Autodesk Inventor part; units mm, degrees
(part 2 of 2)
sketch "Sketch11" plane through (0, 0, 0) normal (0, -1, 0) x (1, 0, 0)
  arc A0 (-20.4663, -10.3703) -> (-20.3393, -10.1987) centre (-21.202, -9.693) ccw projected
  line L0 (-20.4663, -10.3703) -> (-19.459, -11.1159) projected
  arc A1 (-20.4246, -11.8044) -> (-19.459, -11.1159) centre (-21.202, -9.693) ccw projected
  line L1 (-20.4246, -11.8044) -> (-20.8013, -10.6092) projected
  arc A2 (-21.0049, -10.6734) -> (-20.8013, -10.6092) centre (-21.202, -9.693) ccw projected
  line L2 (-21.0049, -10.6734) -> (-20.6282, -11.8686) projected
  arc A3 (-21.8141, -11.8581) -> (-20.6282, -11.8686) centre (-21.202, -9.693) ccw projected
  line L3 (-21.8141, -11.8581) -> (-21.4164, -10.6698) projected
  arc A4 (-21.6188, -10.602) -> (-21.4164, -10.6698) centre (-21.202, -9.693) ccw projected
  line L4 (-21.6188, -10.602) -> (-22.0166, -11.7904) projected
  arc A5 (-22.9699, -11.0848) -> (-22.0166, -11.7904) centre (-21.202, -9.693) ccw projected
  line L5 (-22.9699, -11.0848) -> (-21.9495, -10.3572) projected
  arc A6 (-22.0735, -10.1834) -> (-21.9495, -10.3572) centre (-21.202, -9.693) ccw projected
  line L6 (-22.0735, -10.1834) -> (-23.0938, -10.911) projected
  arc A7 (-23.4503, -9.7799) -> (-23.0938, -10.911) centre (-21.202, -9.693) ccw projected
  line L7 (-23.4503, -9.7799) -> (-22.1972, -9.791) projected
  arc A8 (-22.1953, -9.5775) -> (-22.1972, -9.791) centre (-21.202, -9.693) ccw projected
  line L8 (-22.1953, -9.5775) -> (-23.4484, -9.5664) projected
  arc A9 (-23.072, -8.4418) -> (-23.4484, -9.5664) centre (-21.202, -9.693) ccw projected
  line L9 (-23.072, -8.4418) -> (-22.0647, -9.1873) projected
  arc A10 (-21.9377, -9.0157) -> (-22.0647, -9.1873) centre (-21.202, -9.693) ccw projected
  line L10 (-21.9377, -9.0157) -> (-22.945, -8.2701) projected
  arc A11 (-21.9794, -7.5816) -> (-22.945, -8.2701) centre (-21.202, -9.693) ccw projected
  line L11 (-21.9794, -7.5816) -> (-21.6027, -8.7768) projected
  arc A12 (-21.3991, -8.7126) -> (-21.6027, -8.7768) centre (-21.202, -9.693) ccw projected
  line L12 (-21.3991, -8.7126) -> (-21.7758, -7.5174) projected
  arc A13 (-20.5899, -7.5279) -> (-21.7758, -7.5174) centre (-21.202, -9.693) ccw projected
  line L13 (-20.5899, -7.5279) -> (-20.9876, -8.7162) projected
  arc A14 (-20.7852, -8.784) -> (-20.9876, -8.7162) centre (-21.202, -9.693) ccw projected
  line L14 (-20.7852, -8.784) -> (-20.3874, -7.5956) projected
  arc A15 (-19.4341, -8.3012) -> (-20.3874, -7.5956) centre (-21.202, -9.693) ccw projected
  line L15 (-19.4341, -8.3012) -> (-20.4545, -9.0288) projected
  arc A16 (-20.3305, -9.2026) -> (-20.4545, -9.0288) centre (-21.202, -9.693) ccw projected
  line L16 (-20.3305, -9.2026) -> (-19.3102, -8.475) projected
  arc A17 (-18.9537, -9.6061) -> (-19.3102, -8.475) centre (-21.202, -9.693) ccw projected
  line L17 (-18.9537, -9.6061) -> (-20.2068, -9.595) projected
  arc A18 (-20.2087, -9.8085) -> (-20.2068, -9.595) centre (-21.202, -9.693) ccw projected
  line L18 (-20.2087, -9.8085) -> (-18.9556, -9.8196) projected
  arc A19 (-19.332, -10.9442) -> (-18.9556, -9.8196) centre (-21.202, -9.693) ccw projected
  line L19 (-19.332, -10.9442) -> (-20.3393, -10.1987) projected
  circle A20 centre (0, 28.15) radius 6.2 projected
  arc A21 (20.3393, -10.1987) -> (20.4663, -10.3703) centre (21.202, -9.693) ccw projected
  line L20 (19.332, -10.9442) -> (20.3393, -10.1987) projected
  arc A22 (18.9556, -9.8196) -> (19.332, -10.9442) centre (21.202, -9.693) ccw projected
  line L21 (20.2087, -9.8085) -> (18.9556, -9.8196) projected
  arc A23 (20.2068, -9.595) -> (20.2087, -9.8085) centre (21.202, -9.693) ccw projected
  line L22 (18.9537, -9.6061) -> (20.2068, -9.595) projected
  arc A24 (19.3102, -8.475) -> (18.9537, -9.6061) centre (21.202, -9.693) ccw projected
  line L23 (20.3305, -9.2026) -> (19.3102, -8.475) projected
  arc A25 (20.4545, -9.0288) -> (20.3305, -9.2026) centre (21.202, -9.693) ccw projected
  line L24 (19.4341, -8.3012) -> (20.4545, -9.0288) projected
  arc A26 (20.3874, -7.5956) -> (19.4341, -8.3012) centre (21.202, -9.693) ccw projected
  line L25 (20.7852, -8.784) -> (20.3874, -7.5956) projected
  arc A27 (20.9876, -8.7162) -> (20.7852, -8.784) centre (21.202, -9.693) ccw projected
  line L26 (20.5899, -7.5279) -> (20.9876, -8.7162) projected
  arc A28 (21.7758, -7.5174) -> (20.5899, -7.5279) centre (21.202, -9.693) ccw projected
  line L27 (21.3991, -8.7126) -> (21.7758, -7.5174) projected
  arc A29 (21.6027, -8.7768) -> (21.3991, -8.7126) centre (21.202, -9.693) ccw projected
  line L28 (21.9794, -7.5816) -> (21.6027, -8.7768) projected
  arc A30 (22.945, -8.2701) -> (21.9794, -7.5816) centre (21.202, -9.693) ccw projected
  line L29 (21.9377, -9.0157) -> (22.945, -8.2701) projected
  arc A31 (22.0647, -9.1873) -> (21.9377, -9.0157) centre (21.202, -9.693) ccw projected
  line L30 (23.072, -8.4418) -> (22.0647, -9.1873) projected
  arc A32 (23.4484, -9.5664) -> (23.072, -8.4418) centre (21.202, -9.693) ccw projected
  line L31 (22.1953, -9.5775) -> (23.4484, -9.5664) projected
  arc A33 (22.1972, -9.791) -> (22.1953, -9.5775) centre (21.202, -9.693) ccw projected
  line L32 (23.4503, -9.7799) -> (22.1972, -9.791) projected
  arc A34 (23.0938, -10.911) -> (23.4503, -9.7799) centre (21.202, -9.693) ccw projected
  line L33 (22.0735, -10.1834) -> (23.0938, -10.911) projected
  arc A35 (21.9495, -10.3572) -> (22.0735, -10.1834) centre (21.202, -9.693) ccw projected
  line L34 (22.9699, -11.0848) -> (21.9495, -10.3572) projected
  arc A36 (22.0166, -11.7904) -> (22.9699, -11.0848) centre (21.202, -9.693) ccw projected
  line L35 (21.6188, -10.602) -> (22.0166, -11.7904) projected
  arc A37 (21.4164, -10.6698) -> (21.6188, -10.602) centre (21.202, -9.693) ccw projected
  line L36 (21.8141, -11.8581) -> (21.4164, -10.6698) projected
  arc A38 (20.6282, -11.8686) -> (21.8141, -11.8581) centre (21.202, -9.693) ccw projected
  line L37 (21.0049, -10.6734) -> (20.6282, -11.8686) projected
  arc A39 (20.8013, -10.6092) -> (21.0049, -10.6734) centre (21.202, -9.693) ccw projected
  line L38 (20.4246, -11.8044) -> (20.8013, -10.6092) projected
  arc A40 (19.459, -11.1159) -> (20.4246, -11.8044) centre (21.202, -9.693) ccw projected
  line L39 (20.4663, -10.3703) -> (19.459, -11.1159) projected
  arc A41 (-20.3393, -25.0623) -> (-20.4663, -24.8907) centre (-21.202, -25.568) ccw projected
  line L40 (-19.332, -24.3168) -> (-20.3393, -25.0623) projected
  arc A42 (-18.9556, -25.4414) -> (-19.332, -24.3168) centre (-21.202, -25.568) ccw projected
  line L41 (-20.2087, -25.4525) -> (-18.9556, -25.4414) projected
  arc A43 (-20.2068, -25.666) -> (-20.2087, -25.4525) centre (-21.202, -25.568) ccw projected
  line L42 (-18.9537, -25.6549) -> (-20.2068, -25.666) projected
  arc A44 (-19.3102, -26.786) -> (-18.9537, -25.6549) centre (-21.202, -25.568) ccw projected
  line L43 (-20.3305, -26.0584) -> (-19.3102, -26.786) projected
  arc A45 (-20.4545, -26.2322) -> (-20.3305, -26.0584) centre (-21.202, -25.568) ccw projected
  line L44 (-19.4341, -26.9598) -> (-20.4545, -26.2322) projected
  arc A46 (-20.3874, -27.6654) -> (-19.4341, -26.9598) centre (-21.202, -25.568) ccw projected
  line L45 (-20.7852, -26.477) -> (-20.3874, -27.6654) projected
  arc A47 (-20.9876, -26.5448) -> (-20.7852, -26.477) centre (-21.202, -25.568) ccw projected
  line L46 (-20.5899, -27.7331) -> (-20.9876, -26.5448) projected
  arc A48 (-21.7758, -27.7436) -> (-20.5899, -27.7331) centre (-21.202, -25.568) ccw projected
  line L47 (-21.3991, -26.5484) -> (-21.7758, -27.7436) projected
  arc A49 (-21.6027, -26.4842) -> (-21.3991, -26.5484) centre (-21.202, -25.568) ccw projected
  line L48 (-21.9794, -27.6794) -> (-21.6027, -26.4842) projected
  arc A50 (-22.945, -26.9909) -> (-21.9794, -27.6794) centre (-21.202, -25.568) ccw projected
  line L49 (-21.9377, -26.2453) -> (-22.945, -26.9909) projected
  arc A51 (-22.0647, -26.0737) -> (-21.9377, -26.2453) centre (-21.202, -25.568) ccw projected
  line L50 (-23.072, -26.8192) -> (-22.0647, -26.0737) projected
  arc A52 (-23.4484, -25.6946) -> (-23.072, -26.8192) centre (-21.202, -25.568) ccw projected
  line L51 (-22.1953, -25.6835) -> (-23.4484, -25.6946) projected
  arc A53 (-22.1972, -25.47) -> (-22.1953, -25.6835) centre (-21.202, -25.568) ccw projected
  line L52 (-23.4503, -25.4811) -> (-22.1972, -25.47) projected
  arc A54 (-23.0938, -24.35) -> (-23.4503, -25.4811) centre (-21.202, -25.568) ccw projected
  line L53 (-22.0735, -25.0776) -> (-23.0938, -24.35) projected
  arc A55 (-21.9495, -24.9038) -> (-22.0735, -25.0776) centre (-21.202, -25.568) ccw projected
  line L54 (-22.9699, -24.1762) -> (-21.9495, -24.9038) projected
  arc A56 (-22.0166, -23.4706) -> (-22.9699, -24.1762) centre (-21.202, -25.568) ccw projected
  line L55 (-21.6188, -24.659) -> (-22.0166, -23.4706) projected
  arc A57 (-21.4164, -24.5912) -> (-21.6188, -24.659) centre (-21.202, -25.568) ccw projected
  line L56 (-21.8141, -23.4029) -> (-21.4164, -24.5912) projected
  arc A58 (-20.6282, -23.3924) -> (-21.8141, -23.4029) centre (-21.202, -25.568) ccw projected
  line L57 (-21.0049, -24.5876) -> (-20.6282, -23.3924) projected
  arc A59 (-20.8013, -24.6518) -> (-21.0049, -24.5876) centre (-21.202, -25.568) ccw projected
  line L58 (-20.4246, -23.4566) -> (-20.8013, -24.6518) projected
  arc A60 (-19.459, -24.1451) -> (-20.4246, -23.4566) centre (-21.202, -25.568) ccw projected
  line L59 (-20.4663, -24.8907) -> (-19.459, -24.1451) projected
  circle A61 centre (30.16, -30.16) radius 2.2 projected
  circle A62 centre (-30.16, -30.16) radius 2.2 projected
  line L60 (46.4, 46.4) -> (46.4, -46.4) projected
  line L61 (-46.4, 46.4) -> (46.4, 46.4) projected
  line L62 (-46.4, -46.4) -> (-46.4, 46.4) projected
  line L63 (46.4, -46.4) -> (-46.4, -46.4) projected
  arc A63 (20.4663, -24.8907) -> (20.3393, -25.0623) centre (21.202, -25.568) ccw projected
  line L64 (20.4663, -24.8907) -> (19.459, -24.1451) projected
  arc A64 (20.4246, -23.4566) -> (19.459, -24.1451) centre (21.202, -25.568) ccw projected
  line L65 (20.4246, -23.4566) -> (20.8013, -24.6518) projected
  arc A65 (21.0049, -24.5876) -> (20.8013, -24.6518) centre (21.202, -25.568) ccw projected
  line L66 (21.0049, -24.5876) -> (20.6282, -23.3924) projected
  arc A66 (21.8141, -23.4029) -> (20.6282, -23.3924) centre (21.202, -25.568) ccw projected
  line L67 (21.8141, -23.4029) -> (21.4164, -24.5912) projected
  arc A67 (21.6188, -24.659) -> (21.4164, -24.5912) centre (21.202, -25.568) ccw projected
  line L68 (21.6188, -24.659) -> (22.0166, -23.4706) projected
  arc A68 (22.9699, -24.1762) -> (22.0166, -23.4706) centre (21.202, -25.568) ccw projected
  line L69 (22.9699, -24.1762) -> (21.9495, -24.9038) projected
  arc A69 (22.0735, -25.0776) -> (21.9495, -24.9038) centre (21.202, -25.568) ccw projected
  line L70 (22.0735, -25.0776) -> (23.0938, -24.35) projected
  arc A70 (23.4503, -25.4811) -> (23.0938, -24.35) centre (21.202, -25.568) ccw projected
  line L71 (23.4503, -25.4811) -> (22.1972, -25.47) projected
  arc A71 (22.1953, -25.6835) -> (22.1972, -25.47) centre (21.202, -25.568) ccw projected
  line L72 (22.1953, -25.6835) -> (23.4484, -25.6946) projected
  arc A72 (23.072, -26.8192) -> (23.4484, -25.6946) centre (21.202, -25.568) ccw projected
  line L73 (23.072, -26.8192) -> (22.0647, -26.0737) projected
  arc A73 (21.9377, -26.2453) -> (22.0647, -26.0737) centre (21.202, -25.568) ccw projected
  line L74 (21.9377, -26.2453) -> (22.945, -26.9909) projected
  arc A74 (21.9794, -27.6794) -> (22.945, -26.9909) centre (21.202, -25.568) ccw projected
  line L75 (21.9794, -27.6794) -> (21.6027, -26.4842) projected
  arc A75 (21.3991, -26.5484) -> (21.6027, -26.4842) centre (21.202, -25.568) ccw projected
  line L76 (21.3991, -26.5484) -> (21.7758, -27.7436) projected
  arc A76 (20.5899, -27.7331) -> (21.7758, -27.7436) centre (21.202, -25.568) ccw projected
  line L77 (20.5899, -27.7331) -> (20.9876, -26.5448) projected
  arc A77 (20.7852, -26.477) -> (20.9876, -26.5448) centre (21.202, -25.568) ccw projected
  line L78 (20.7852, -26.477) -> (20.3874, -27.6654) projected
  arc A78 (19.4341, -26.9598) -> (20.3874, -27.6654) centre (21.202, -25.568) ccw projected
  line L79 (19.4341, -26.9598) -> (20.4545, -26.2322) projected
  arc A79 (20.3305, -26.0584) -> (20.4545, -26.2322) centre (21.202, -25.568) ccw projected
  line L80 (20.3305, -26.0584) -> (19.3102, -26.786) projected
  arc A80 (18.9537, -25.6549) -> (19.3102, -26.786) centre (21.202, -25.568) ccw projected
  line L81 (18.9537, -25.6549) -> (20.2068, -25.666) projected
  arc A81 (20.2087, -25.4525) -> (20.2068, -25.666) centre (21.202, -25.568) ccw projected
  line L82 (20.2087, -25.4525) -> (18.9556, -25.4414) projected
  arc A82 (19.332, -24.3168) -> (18.9556, -25.4414) centre (21.202, -25.568) ccw projected
  line L83 (19.332, -24.3168) -> (20.3393, -25.0623) projected
  line L84 (-16.702, 14.187) -> (16.702, 14.187) construction
  line L85 (-16.702, -36.813) -> (-16.702, 14.187) construction
  line L86 (16.702, -36.813) -> (16.702, 14.187) construction
  arc A83 (-20.4663, -10.3703) -> (-20.3393, -10.1987) centre (-21.202, -9.693) ccw construction
  line L87 (-20.4663, -10.3703) -> (-19.459, -11.1159) construction
  arc A84 (-20.4246, -11.8044) -> (-19.459, -11.1159) centre (-21.202, -9.693) ccw construction
  line L88 (-20.4246, -11.8044) -> (-20.8013, -10.6092) construction
  arc A85 (-21.0049, -10.6734) -> (-20.8013, -10.6092) centre (-21.202, -9.693) ccw construction
  line L89 (-21.0049, -10.6734) -> (-20.6282, -11.8686) construction
  arc A86 (-21.8141, -11.8581) -> (-20.6282, -11.8686) centre (-21.202, -9.693) ccw construction
  line L90 (-21.8141, -11.8581) -> (-21.4164, -10.6698) construction
  arc A87 (-21.6188, -10.602) -> (-21.4164, -10.6698) centre (-21.202, -9.693) ccw construction
  line L91 (-21.6188, -10.602) -> (-22.0166, -11.7904) construction
  arc A88 (-22.9699, -11.0848) -> (-22.0166, -11.7904) centre (-21.202, -9.693) ccw construction
  line L92 (-22.9699, -11.0848) -> (-21.9495, -10.3572) construction
  arc A89 (-22.0735, -10.1834) -> (-21.9495, -10.3572) centre (-21.202, -9.693) ccw construction
  line L93 (-22.0735, -10.1834) -> (-23.0938, -10.911) construction
  arc A90 (-23.4503, -9.7799) -> (-23.0938, -10.911) centre (-21.202, -9.693) ccw construction
  line L94 (-23.4503, -9.7799) -> (-22.1972, -9.791) construction
  arc A91 (-22.1953, -9.5775) -> (-22.1972, -9.791) centre (-21.202, -9.693) ccw construction
  line L95 (-22.1953, -9.5775) -> (-23.4484, -9.5664) construction
  arc A92 (-23.072, -8.4418) -> (-23.4484, -9.5664) centre (-21.202, -9.693) ccw construction
  line L96 (-23.072, -8.4418) -> (-22.0647, -9.1873) construction
  arc A93 (-21.9377, -9.0157) -> (-22.0647, -9.1873) centre (-21.202, -9.693) ccw construction
  line L97 (-21.9377, -9.0157) -> (-22.945, -8.2701) construction
  arc A94 (-21.9794, -7.5816) -> (-22.945, -8.2701) centre (-21.202, -9.693) ccw construction
  line L98 (-21.9794, -7.5816) -> (-21.6027, -8.7768) construction
  arc A95 (-21.3991, -8.7126) -> (-21.6027, -8.7768) centre (-21.202, -9.693) ccw construction
  line L99 (-21.3991, -8.7126) -> (-21.7758, -7.5174) construction
  arc A96 (-20.5899, -7.5279) -> (-21.7758, -7.5174) centre (-21.202, -9.693) ccw construction
  line L100 (-20.5899, -7.5279) -> (-20.9876, -8.7162) construction
  arc A97 (-20.7852, -8.784) -> (-20.9876, -8.7162) centre (-21.202, -9.693) ccw construction
  line L101 (-20.7852, -8.784) -> (-20.3874, -7.5956) construction
  arc A98 (-19.4341, -8.3012) -> (-20.3874, -7.5956) centre (-21.202, -9.693) ccw construction
  line L102 (-19.4341, -8.3012) -> (-20.4545, -9.0288) construction
  arc A99 (-20.3305, -9.2026) -> (-20.4545, -9.0288) centre (-21.202, -9.693) ccw construction
  line L103 (-20.3305, -9.2026) -> (-19.3102, -8.475) construction
  arc A100 (-18.9537, -9.6061) -> (-19.3102, -8.475) centre (-21.202, -9.693) ccw construction
  line L104 (-18.9537, -9.6061) -> (-20.2068, -9.595) construction
  arc A101 (-20.2087, -9.8085) -> (-20.2068, -9.595) centre (-21.202, -9.693) ccw construction
  line L105 (-20.2087, -9.8085) -> (-18.9556, -9.8196) construction
  arc A102 (-19.332, -10.9442) -> (-18.9556, -9.8196) centre (-21.202, -9.693) ccw construction
  line L106 (-19.332, -10.9442) -> (-20.3393, -10.1987) construction
  circle A103 centre (0, 28.15) radius 6.2 construction
  arc A104 (20.3393, -10.1987) -> (20.4663, -10.3703) centre (21.202, -9.693) ccw construction
  line L107 (19.332, -10.9442) -> (20.3393, -10.1987) construction
  arc A105 (18.9556, -9.8196) -> (19.332, -10.9442) centre (21.202, -9.693) ccw construction
  line L108 (20.2087, -9.8085) -> (18.9556, -9.8196) construction
  arc A106 (20.2068, -9.595) -> (20.2087, -9.8085) centre (21.202, -9.693) ccw construction
  line L109 (18.9537, -9.6061) -> (20.2068, -9.595) construction
  arc A107 (19.3102, -8.475) -> (18.9537, -9.6061) centre (21.202, -9.693) ccw construction
  line L110 (20.3305, -9.2026) -> (19.3102, -8.475) construction
  arc A108 (20.4545, -9.0288) -> (20.3305, -9.2026) centre (21.202, -9.693) ccw construction
  line L111 (19.4341, -8.3012) -> (20.4545, -9.0288) construction
  arc A109 (20.3874, -7.5956) -> (19.4341, -8.3012) centre (21.202, -9.693) ccw construction
  line L112 (20.7852, -8.784) -> (20.3874, -7.5956) construction
  arc A110 (20.9876, -8.7162) -> (20.7852, -8.784) centre (21.202, -9.693) ccw construction
  line L113 (20.5899, -7.5279) -> (20.9876, -8.7162) construction
  arc A111 (21.7758, -7.5174) -> (20.5899, -7.5279) centre (21.202, -9.693) ccw construction
  line L114 (21.3991, -8.7126) -> (21.7758, -7.5174) construction
  arc A112 (21.6027, -8.7768) -> (21.3991, -8.7126) centre (21.202, -9.693) ccw construction
  line L115 (21.9794, -7.5816) -> (21.6027, -8.7768) construction
  arc A113 (22.945, -8.2701) -> (21.9794, -7.5816) centre (21.202, -9.693) ccw construction
  line L116 (21.9377, -9.0157) -> (22.945, -8.2701) construction
  arc A114 (22.0647, -9.1873) -> (21.9377, -9.0157) centre (21.202, -9.693) ccw construction
  line L117 (23.072, -8.4418) -> (22.0647, -9.1873) construction
  arc A115 (23.4484, -9.5664) -> (23.072, -8.4418) centre (21.202, -9.693) ccw construction
  line L118 (22.1953, -9.5775) -> (23.4484, -9.5664) construction
  arc A116 (22.1972, -9.791) -> (22.1953, -9.5775) centre (21.202, -9.693) ccw construction
  line L119 (23.4503, -9.7799) -> (22.1972, -9.791) construction
  arc A117 (23.0938, -10.911) -> (23.4503, -9.7799) centre (21.202, -9.693) ccw construction
  line L120 (22.0735, -10.1834) -> (23.0938, -10.911) construction
  arc A118 (21.9495, -10.3572) -> (22.0735, -10.1834) centre (21.202, -9.693) ccw construction
  line L121 (22.9699, -11.0848) -> (21.9495, -10.3572) construction
  arc A119 (22.0166, -11.7904) -> (22.9699, -11.0848) centre (21.202, -9.693) ccw construction
  line L122 (21.6188, -10.602) -> (22.0166, -11.7904) construction
  arc A120 (21.4164, -10.6698) -> (21.6188, -10.602) centre (21.202, -9.693) ccw construction
  line L123 (21.8141, -11.8581) -> (21.4164, -10.6698) construction
  arc A121 (20.6282, -11.8686) -> (21.8141, -11.8581) centre (21.202, -9.693) ccw construction
  line L124 (21.0049, -10.6734) -> (20.6282, -11.8686) construction
  arc A122 (20.8013, -10.6092) -> (21.0049, -10.6734) centre (21.202, -9.693) ccw construction
  line L125 (20.4246, -11.8044) -> (20.8013, -10.6092) construction
  arc A123 (19.459, -11.1159) -> (20.4246, -11.8044) centre (21.202, -9.693) ccw construction
  line L126 (20.4663, -10.3703) -> (19.459, -11.1159) construction
  arc A124 (-20.3393, -25.0623) -> (-20.4663, -24.8907) centre (-21.202, -25.568) ccw construction
  line L127 (-19.332, -24.3168) -> (-20.3393, -25.0623) construction
  arc A125 (-18.9556, -25.4414) -> (-19.332, -24.3168) centre (-21.202, -25.568) ccw construction
  line L128 (-20.2087, -25.4525) -> (-18.9556, -25.4414) construction
  arc A126 (-20.2068, -25.666) -> (-20.2087, -25.4525) centre (-21.202, -25.568) ccw construction
  line L129 (-18.9537, -25.6549) -> (-20.2068, -25.666) construction
  arc A127 (-19.3102, -26.786) -> (-18.9537, -25.6549) centre (-21.202, -25.568) ccw construction
  line L130 (-20.3305, -26.0584) -> (-19.3102, -26.786) construction
  arc A128 (-20.4545, -26.2322) -> (-20.3305, -26.0584) centre (-21.202, -25.568) ccw construction
  line L131 (-19.4341, -26.9598) -> (-20.4545, -26.2322) construction
  arc A129 (-20.3874, -27.6654) -> (-19.4341, -26.9598) centre (-21.202, -25.568) ccw construction
  line L132 (-20.7852, -26.477) -> (-20.3874, -27.6654) construction
  arc A130 (-20.9876, -26.5448) -> (-20.7852, -26.477) centre (-21.202, -25.568) ccw construction
  line L133 (-20.5899, -27.7331) -> (-20.9876, -26.5448) construction
  arc A131 (-21.7758, -27.7436) -> (-20.5899, -27.7331) centre (-21.202, -25.568) ccw construction
  line L134 (-21.3991, -26.5484) -> (-21.7758, -27.7436) construction
  arc A132 (-21.6027, -26.4842) -> (-21.3991, -26.5484) centre (-21.202, -25.568) ccw construction
  line L135 (-21.9794, -27.6794) -> (-21.6027, -26.4842) construction
  arc A133 (-22.945, -26.9909) -> (-21.9794, -27.6794) centre (-21.202, -25.568) ccw construction
  line L136 (-21.9377, -26.2453) -> (-22.945, -26.9909) construction
  arc A134 (-22.0647, -26.0737) -> (-21.9377, -26.2453) centre (-21.202, -25.568) ccw construction
  line L137 (-23.072, -26.8192) -> (-22.0647, -26.0737) construction
  arc A135 (-23.4484, -25.6946) -> (-23.072, -26.8192) centre (-21.202, -25.568) ccw construction
  line L138 (-22.1953, -25.6835) -> (-23.4484, -25.6946) construction
  arc A136 (-22.1972, -25.47) -> (-22.1953, -25.6835) centre (-21.202, -25.568) ccw construction
  line L139 (-23.4503, -25.4811) -> (-22.1972, -25.47) construction
  arc A137 (-23.0938, -24.35) -> (-23.4503, -25.4811) centre (-21.202, -25.568) ccw construction
  line L140 (-22.0735, -25.0776) -> (-23.0938, -24.35) construction
  arc A138 (-21.9495, -24.9038) -> (-22.0735, -25.0776) centre (-21.202, -25.568) ccw construction
  line L141 (-22.9699, -24.1762) -> (-21.9495, -24.9038) construction
  arc A139 (-22.0166, -23.4706) -> (-22.9699, -24.1762) centre (-21.202, -25.568) ccw construction
  line L142 (-21.6188, -24.659) -> (-22.0166, -23.4706) construction
  arc A140 (-21.4164, -24.5912) -> (-21.6188, -24.659) centre (-21.202, -25.568) ccw construction
  line L143 (-21.8141, -23.4029) -> (-21.4164, -24.5912) construction
  arc A141 (-20.6282, -23.3924) -> (-21.8141, -23.4029) centre (-21.202, -25.568) ccw construction
  line L144 (-21.0049, -24.5876) -> (-20.6282, -23.3924) construction
  arc A142 (-20.8013, -24.6518) -> (-21.0049, -24.5876) centre (-21.202, -25.568) ccw construction
  line L145 (-20.4246, -23.4566) -> (-20.8013, -24.6518) construction
  arc A143 (-19.459, -24.1451) -> (-20.4246, -23.4566) centre (-21.202, -25.568) ccw construction
  line L146 (-20.4663, -24.8907) -> (-19.459, -24.1451) construction
  circle A144 centre (30.16, -30.16) radius 2.2 construction
  circle A145 centre (-30.16, -30.16) radius 2.2 construction
  line L147 (46.4, 46.4) -> (46.4, -46.4) construction
  line L148 (-46.4, 46.4) -> (46.4, 46.4) construction
  line L149 (-46.4, -46.4) -> (-46.4, 46.4) construction
  line L150 (46.4, -46.4) -> (-46.4, -46.4) construction
  arc A146 (20.4663, -24.8907) -> (20.3393, -25.0623) centre (21.202, -25.568) ccw construction
  line L151 (20.4663, -24.8907) -> (19.459, -24.1451) construction
  arc A147 (20.4246, -23.4566) -> (19.459, -24.1451) centre (21.202, -25.568) ccw construction
  line L152 (20.4246, -23.4566) -> (20.8013, -24.6518) construction
  arc A148 (21.0049, -24.5876) -> (20.8013, -24.6518) centre (21.202, -25.568) ccw construction
  line L153 (21.0049, -24.5876) -> (20.6282, -23.3924) construction
  arc A149 (21.8141, -23.4029) -> (20.6282, -23.3924) centre (21.202, -25.568) ccw construction
  line L154 (21.8141, -23.4029) -> (21.4164, -24.5912) construction
  arc A150 (21.6188, -24.659) -> (21.4164, -24.5912) centre (21.202, -25.568) ccw construction
  line L155 (21.6188, -24.659) -> (22.0166, -23.4706) construction
  arc A151 (22.9699, -24.1762) -> (22.0166, -23.4706) centre (21.202, -25.568) ccw construction
  line L156 (22.9699, -24.1762) -> (21.9495, -24.9038) construction
  arc A152 (22.0735, -25.0776) -> (21.9495, -24.9038) centre (21.202, -25.568) ccw construction
  line L157 (22.0735, -25.0776) -> (23.0938, -24.35) construction
  arc A153 (23.4503, -25.4811) -> (23.0938, -24.35) centre (21.202, -25.568) ccw construction
  line L158 (23.4503, -25.4811) -> (22.1972, -25.47) construction
  arc A154 (22.1953, -25.6835) -> (22.1972, -25.47) centre (21.202, -25.568) ccw construction
  line L159 (22.1953, -25.6835) -> (23.4484, -25.6946) construction
  arc A155 (23.072, -26.8192) -> (23.4484, -25.6946) centre (21.202, -25.568) ccw construction
  line L160 (23.072, -26.8192) -> (22.0647, -26.0737) construction
  arc A156 (21.9377, -26.2453) -> (22.0647, -26.0737) centre (21.202, -25.568) ccw construction
  line L161 (21.9377, -26.2453) -> (22.945, -26.9909) construction
  arc A157 (21.9794, -27.6794) -> (22.945, -26.9909) centre (21.202, -25.568) ccw construction
  line L162 (21.9794, -27.6794) -> (21.6027, -26.4842) construction
  arc A158 (21.3991, -26.5484) -> (21.6027, -26.4842) centre (21.202, -25.568) ccw construction
  line L163 (21.3991, -26.5484) -> (21.7758, -27.7436) construction
  arc A159 (20.5899, -27.7331) -> (21.7758, -27.7436) centre (21.202, -25.568) ccw construction
  line L164 (20.5899, -27.7331) -> (20.9876, -26.5448) construction
  arc A160 (20.7852, -26.477) -> (20.9876, -26.5448) centre (21.202, -25.568) ccw construction
  line L165 (20.7852, -26.477) -> (20.3874, -27.6654) construction
  arc A161 (19.4341, -26.9598) -> (20.3874, -27.6654) centre (21.202, -25.568) ccw construction
  line L166 (19.4341, -26.9598) -> (20.4545, -26.2322) construction
  arc A162 (20.3305, -26.0584) -> (20.4545, -26.2322) centre (21.202, -25.568) ccw construction
  line L167 (20.3305, -26.0584) -> (19.3102, -26.786) construction
  arc A163 (18.9537, -25.6549) -> (19.3102, -26.786) centre (21.202, -25.568) ccw construction
  line L168 (18.9537, -25.6549) -> (20.2068, -25.666) construction
  arc A164 (20.2087, -25.4525) -> (20.2068, -25.666) centre (21.202, -25.568) ccw construction
  line L169 (20.2087, -25.4525) -> (18.9556, -25.4414) construction
  arc A165 (19.332, -24.3168) -> (18.9556, -25.4414) centre (21.202, -25.568) ccw construction
  line L170 (19.332, -24.3168) -> (20.3393, -25.0623) construction
  line L171 (0, 18.2733) -> (-16.702, 18.2733) construction
  line L172 (-16.702, 18.2733) -> (-16.702, 14.187) construction
  line L173 (16.702, 14.187) -> (-16.702, 18.2733) construction
  line L174 (0, 18.2733) -> (16.702, 18.2733) construction
  line L175 (-16.702, 14.187) -> (16.702, 18.2733) construction
  line L176 (16.702, 14.187) -> (16.702, 18.2733) construction
  line L177 (0, 16.2301) -> (-16.702, 16.2301) construction
  circle A166 centre (-14.0927, 16.2301) radius 1
  point P0 (0, 0)
  dimension "d81" = 2
  constraints: 14 end point, 2 horizontal, 2 midpoint, 1 centre point, 1 parallel, 1 perpendicular, 1 point on line, 1 vertical
  measures "d81" diameter of A166
extrude "Extrusion13" cut sketch "Sketch11" against normal blind 10 contours A166
mirror "Mirror10" about plane through (0, 0, -46.4) normal (-1, 0, 0) of "Extrusion13"
sketch "Sketch14" plane through (0, 5, 0) normal (0, 1, 0) x (1, 0, 0)
  line L0 (-46.4, 41.4) -> (-46.4, -41.4) projected
  line L1 (-46.4, 0) -> (-46.4, -10)
  line L2 (-46.4, -10) -> (-38.9, -10)
  line L3 (-38.9, -10) -> (-38.9, 10)
  line L4 (-38.9, 10) -> (-46.4, 10)
  line L5 (-46.4, 0) -> (-46.4, 10)
  line L6 (-39.5, 9.4) -> (-39.5, -9.4)
  line L7 (-39.5, -9.4) -> (-45.8, -9.4)
  line L8 (-45.8, -9.4) -> (-45.8, 0)
  line L9 (-45.8, 0) -> (-45.8, 9.4)
  line L10 (-45.8, 9.4) -> (-39.5, 9.4)
  line L11 (-42.4, -46.4) -> (42.4, -46.4) construction
  line L12 (0, -46.4) -> (-20, -46.4) construction
  line L13 (-20, -46.4) -> (-20, -38.9)
  line L14 (-20, -38.9) -> (-40, -38.9)
  line L15 (-40, -38.9) -> (-40, -46.4)
  line L16 (-40, -46.4) -> (-20, -46.4)
  line L17 (-39.4, -45.8) -> (-39.4, -39.5)
  line L18 (-39.4, -39.5) -> (-20.6, -39.5)
  line L19 (-20.6, -39.5) -> (-20.6, -45.8)
  line L20 (-20.6, -45.8) -> (-39.4, -45.8)
  point P0 (0, 0)
  dimension "d90" = 10
  dimension "d91" = 7.5
  dimension "d92" = 20
  dimension "d93" = 0.6
  dimension "d94" = 20
  dimension "d95" = 7.5
  dimension "d96" = 20
  dimension "d97" = 0.6
  constraints: 38 end point, 11 perpendicular, 4 point on line, 2 collinear, 2 midpoint, 7 other
  measures "d90" distance of L1.start L1.end
  measures "d91" distance of L1.end L2.end
  measures "d92" distance of L2.end L3.end
  measures "d93" distance between parallel lines of L3 L6
  measures "d94" distance of L12.start L12.end
  measures "d95" distance of L12.end L13.end
  measures "d96" distance of L13.end L14.end
  measures "d97" distance between parallel lines of L15 L17
extrude "Extrusion16" add sketch "Sketch14" along normal blind 6
mirror "Mirror14" about plane through (0, 0, -46.4) normal (-1, 0, 0) of "Extrusion16"
mirror "Mirror15" about plane through (-46.4, 0, 0) normal (0, 0, 1) of "Extrusion16", "Mirror14"
ref_plane "Work Plane8" through (0, 0, -46.4) normal (-1, 0, 0) x (0, 0, 1)
ref_plane "Work Plane9" through (0, 0, 46.4) normal (1, 0, 0) x (0, 0, -1)
ref_plane "Work Plane10" through (0, 0, 46.4) normal (1, 0, 0) x (0, 0, -1)
body "Solid1"
